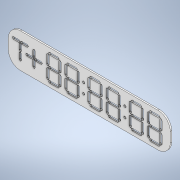
# Autodesk Inventor part: 7 Segment Clock
Saved by Autodesk Inventor 2021 (Build 250183000, 183)
## iProperties
Created: 2020-06-26
Part Number: 7 Segment Clock
Material: White
Document SubType Name: Modeling
Designer: dech3
Density: 1.188 g/cm^3
Appearance: Polycarbonate - Clear
Author: dech3
Autodesk Inventor part; units mm, degrees
(part 1 of 3)
ref_plane "YZ Plane" through (0, 0, 0) normal (1, 0, 0) x (0, 1, 0)
ref_plane "XZ Plane" through (0, 0, 0) normal (0, 1, 0) x (-1, 0, 0)
ref_plane "XY Plane" through (0, 0, 0) normal (0, 0, 1) x (1, 0, 0)
sketch "Single Segment" plane through (0, 0, 0) normal (0, 0, 1) x (1, 0, 0)
  arc A0 (128.9839, -2.0293) -> (129.691, -2.3222) centre (129.691, -1.3222) ccw
  arc A1 (129.691, 2.6778) -> (128.9839, 2.3849) centre (129.691, 1.6778) ccw
  line L0 (128.9839, -2.0293) -> (127.0768, -0.1222)
  line L1 (128.9839, 2.3849) -> (127.0768, 0.4778)
  line L2 (127.0768, 0.1778) -> (127.0768, -0.1222)
  line L3 (127.0768, 0.1778) -> (127.0768, 0.4778)
  line L4 (129.691, 2.6778) -> (146.4626, 2.6778)
  line L5 (146.4626, -2.3222) -> (129.691, -2.3222)
  arc A2 (147.1697, 2.3849) -> (146.4626, 2.6778) centre (146.4626, 1.6778) ccw
  line L6 (147.1697, 2.3849) -> (149.0768, 0.4778)
  line L7 (149.0768, 0.1778) -> (149.0768, 0.4778)
  line L8 (149.0768, 0.1778) -> (149.0768, -0.1222)
  arc A3 (146.4626, -2.3222) -> (147.1697, -2.0293) centre (146.4626, -1.3222) ccw
  line L9 (147.1697, -2.0293) -> (149.0768, -0.1222)
  point P0 (153.0768, 0)
  point P1 (129.2768, -2.3222)
  point P2 (129.2768, 2.6778)
  point P3 (146.8768, 2.6778)
  point P4 (146.8768, -2.3222)
  dimension "d105" = 2.2
  dimension "d108" = 2.2
  dimension "d111" = 2.2
  dimension "d112" = 2.2
  dimension "d113" = 2.2
  dimension "d114" = 2.2
  dimension "d115" = 2.2
  dimension "d116" = 1
  dimension "d117" = 5
  dimension "d121" = 2.2
  dimension "d122" = 2.2
  dimension "d126" = 135
  dimension "d127" = 22
  dimension "d128" = 135
  dimension "d129" = 2.5
  dimension "d348" = 5
  dimension "d349" = 22
  dimension "d350" = 2.2
  dimension "d352" = 0.3
  dimension "d353" = 0.3
  dimension "d358" = 0.3
  dimension "d359" = 0.3
  measures "d105" horizontal distance of point (129.277, -2.322) L0.end
  measures "d108" horizontal distance of L7.end point (146.877, 2.678)
  measures "d111" horizontal distance of point (129.277, 2.678) L3.end
  measures "d112" horizontal distance of L9.end point (146.877, -2.322)
  measures "d113" horizontal distance of L9.end point (146.877, -2.322)
  measures "d114" horizontal distance of point (129.277, 2.678) L3.end
  measures "d115" horizontal distance of point (129.277, -2.322) L0.end
  measures "d116" radius of A1
  measures "d117" distance of point (146.877, -2.322) point (146.877, 2.678)
  measures "d121" horizontal distance of L7.end point (146.877, 2.678)
  measures "d122" horizontal distance of point (146.877, -2.322) L8.start
  measures "d126" angle of L5 L9
  measures "d127" horizontal distance of L9.end L3.start
  measures "d128" angle of L4 L6
  measures "d129" vertical distance of L8.start point (146.877, -2.322)
  measures "d348" distance between parallel lines of L5 L4
  measures "d349" distance of L3.start L8.start
  measures "d350" horizontal distance of point (129.277, 2.678) L3.start
  measures "d352" distance of L8.start L7.end
  measures "d353" distance of L9.end L8.start
  measures "d358" distance of L3.end L3.start
  measures "d359" distance of L0.end L3.start
sketch "7 Segment Digit" plane through (0, 0, 0) normal (0, 0, 1) x (1, 0, 0)
  arc A0 (215.9071, -11.0293) -> (216.6142, -11.3222) centre (216.6142, -10.3222) ccw
  arc A1 (216.6142, -6.3222) -> (215.9071, -6.6151) centre (216.6142, -7.3222) ccw
  line L0 (215.9071, -11.0293) -> (214, -9.1222)
  line L1 (215.9071, -6.6151) -> (214, -8.5222)
  line L2 (214, -8.8222) -> (214, -9.1222)
  line L3 (214, -8.8222) -> (214, -8.5222)
  line L4 (216.6142, -6.3222) -> (233.3858, -6.3222)
  line L5 (233.3858, -11.3222) -> (216.6142, -11.3222)
  arc A2 (234.0929, -6.6151) -> (233.3858, -6.3222) centre (233.3858, -7.3222) ccw
  line L6 (234.0929, -6.6151) -> (236, -8.5222)
  line L7 (236, -8.8222) -> (236, -8.5222)
  line L8 (236, -8.8222) -> (236, -9.1222)
  arc A3 (233.3858, -11.3222) -> (234.0929, -11.0293) centre (233.3858, -10.3222) ccw
  line L9 (234.0929, -11.0293) -> (236, -9.1222)
  arc A4 (215.9071, -35.8293) -> (216.6142, -36.1222) centre (216.6142, -35.1222) ccw
  arc A5 (216.6142, -31.1222) -> (215.9071, -31.4151) centre (216.6142, -32.1222) ccw
  line L10 (215.9071, -35.8293) -> (214, -33.9222)
  line L11 (215.9071, -31.4151) -> (214, -33.3222)
  line L12 (214, -33.6222) -> (214, -33.9222)
  line L13 (214, -33.6222) -> (214, -33.3222)
  line L14 (216.6142, -31.1222) -> (233.3858, -31.1222)
  line L15 (233.3858, -36.1222) -> (216.6142, -36.1222)
  arc A6 (234.0929, -31.4151) -> (233.3858, -31.1222) centre (233.3858, -32.1222) ccw
  line L16 (234.0929, -31.4151) -> (236, -33.3222)
  line L17 (236, -33.6222) -> (236, -33.3222)
  line L18 (236, -33.6222) -> (236, -33.9222)
  arc A7 (233.3858, -36.1222) -> (234.0929, -35.8293) centre (233.3858, -35.1222) ccw
  line L19 (234.0929, -35.8293) -> (236, -33.9222)
  arc A8 (214.8071, -30.3151) -> (215.1, -29.608) centre (214.1, -29.608) ccw
  arc A9 (210.1, -29.608) -> (210.3929, -30.3151) centre (211.1, -29.608) ccw
  line L20 (214.8071, -30.3151) -> (212.9, -32.2222)
  line L21 (210.3929, -30.3151) -> (212.3, -32.2222)
  line L22 (212.6, -32.2222) -> (212.9, -32.2222)
  line L23 (212.6, -32.2222) -> (212.3, -32.2222)
  line L24 (210.1, -29.608) -> (210.1, -12.8364)
  line L25 (215.1, -12.8364) -> (215.1, -29.608)
  arc A10 (210.3929, -12.1293) -> (210.1, -12.8364) centre (211.1, -12.8364) ccw
  line L26 (210.3929, -12.1293) -> (212.3, -10.2222)
  line L27 (212.6, -10.2222) -> (212.3, -10.2222)
  line L28 (212.6, -10.2222) -> (212.9, -10.2222)
  arc A11 (215.1, -12.8364) -> (214.8071, -12.1293) centre (214.1, -12.8364) ccw
  line L29 (214.8071, -12.1293) -> (212.9, -10.2222)
  arc A12 (214.8071, -55.1151) -> (215.1, -54.408) centre (214.1, -54.408) ccw
  arc A13 (210.1, -54.408) -> (210.3929, -55.1151) centre (211.1, -54.408) ccw
  line L30 (214.8071, -55.1151) -> (212.9, -57.0222)
  line L31 (210.3929, -55.1151) -> (212.3, -57.0222)
  line L32 (212.6, -57.0222) -> (212.9, -57.0222)
  line L33 (212.6, -57.0222) -> (212.3, -57.0222)
  line L34 (210.1, -54.408) -> (210.1, -37.6364)
  line L35 (215.1, -37.6364) -> (215.1, -54.408)
  arc A14 (210.3929, -36.9293) -> (210.1, -37.6364) centre (211.1, -37.6364) ccw
  line L36 (210.3929, -36.9293) -> (212.3, -35.0222)
  line L37 (212.6, -35.0222) -> (212.3, -35.0222)
  line L38 (212.6, -35.0222) -> (212.9, -35.0222)
  arc A15 (215.1, -37.6364) -> (214.8071, -36.9293) centre (214.1, -37.6364) ccw
  line L39 (214.8071, -36.9293) -> (212.9, -35.0222)
  arc A16 (239.6071, -30.3151) -> (239.9, -29.608) centre (238.9, -29.608) ccw
  arc A17 (234.9, -29.608) -> (235.1929, -30.3151) centre (235.9, -29.608) ccw
  line L40 (239.6071, -30.3151) -> (237.7, -32.2222)
  line L41 (235.1929, -30.3151) -> (237.1, -32.2222)
  line L42 (237.4, -32.2222) -> (237.7, -32.2222)
  line L43 (237.4, -32.2222) -> (237.1, -32.2222)
  line L44 (234.9, -29.608) -> (234.9, -12.8364)
  line L45 (239.9, -12.8364) -> (239.9, -29.608)
  arc A18 (235.1929, -12.1293) -> (234.9, -12.8364) centre (235.9, -12.8364) ccw
  line L46 (235.1929, -12.1293) -> (237.1, -10.2222)
  line L47 (237.4, -10.2222) -> (237.1, -10.2222)
  line L48 (237.4, -10.2222) -> (237.7, -10.2222)
  arc A19 (239.9, -12.8364) -> (239.6071, -12.1293) centre (238.9, -12.8364) ccw
  line L49 (239.6071, -12.1293) -> (237.7, -10.2222)
  arc A20 (239.6071, -55.1151) -> (239.9, -54.408) centre (238.9, -54.408) ccw
  arc A21 (234.9, -54.408) -> (235.1929, -55.1151) centre (235.9, -54.408) ccw
  line L50 (239.6071, -55.1151) -> (237.7, -57.0222)
  line L51 (235.1929, -55.1151) -> (237.1, -57.0222)
  line L52 (237.4, -57.0222) -> (237.7, -57.0222)
  line L53 (237.4, -57.0222) -> (237.1, -57.0222)
  line L54 (234.9, -54.408) -> (234.9, -37.6364)
  line L55 (239.9, -37.6364) -> (239.9, -54.408)
  arc A22 (235.1929, -36.9293) -> (234.9, -37.6364) centre (235.9, -37.6364) ccw
  line L56 (235.1929, -36.9293) -> (237.1, -35.0222)
  line L57 (237.4, -35.0222) -> (237.1, -35.0222)
  line L58 (237.4, -35.0222) -> (237.7, -35.0222)
  arc A23 (239.9, -37.6364) -> (239.6071, -36.9293) centre (238.9, -37.6364) ccw
  line L59 (239.6071, -36.9293) -> (237.7, -35.0222)
  arc A24 (215.9071, -60.6293) -> (216.6142, -60.9222) centre (216.6142, -59.9222) ccw
  arc A25 (216.6142, -55.9222) -> (215.9071, -56.2151) centre (216.6142, -56.9222) ccw
  line L60 (215.9071, -60.6293) -> (214, -58.7222)
  line L61 (215.9071, -56.2151) -> (214, -58.1222)
  line L62 (214, -58.4222) -> (214, -58.7222)
  line L63 (214, -58.4222) -> (214, -58.1222)
  line L64 (216.6142, -55.9222) -> (233.3858, -55.9222)
  line L65 (233.3858, -60.9222) -> (216.6142, -60.9222)
  arc A26 (234.0929, -56.2151) -> (233.3858, -55.9222) centre (233.3858, -56.9222) ccw
  line L66 (234.0929, -56.2151) -> (236, -58.1222)
  line L67 (236, -58.4222) -> (236, -58.1222)
  line L68 (236, -58.4222) -> (236, -58.7222)
  arc A27 (233.3858, -60.9222) -> (234.0929, -60.6293) centre (233.3858, -59.9222) ccw
  line L69 (234.0929, -60.6293) -> (236, -58.7222)
  point P0 (239.8857, -4.9143)
  dimension "d131" = 1.1
  dimension "d132" = 1.1
  dimension "d137" = 1.1
  dimension "d138" = 1.1
  dimension "d139" = 1.1
  dimension "d140" = 1.1
  dimension "d141" = 1.1
  dimension "d142" = 1.1
  dimension "d143" = 1.1
  dimension "d144" = 1.1
  dimension "d145" = 1.1
  dimension "d146" = 1.1
  dimension "d150" = 1.1
  dimension "d151" = 1.1
  dimension "d152" = 1.1
  dimension "d153" = 1.1
sketch "Slanted Segment Large" plane through (0, 0, 0) normal (0, 0, 1) x (1, 0, 0)
  line L0 (-252.8296, -124.6537) -> (-254.4296, -124.6537)
  line L1 (-254.4296, -124.6537) -> (-257.6296, -127.8537)
  line L2 (-257.6296, -127.8537) -> (-261.6917, -184.8537)
  line L3 (-253.6917, -184.8537) -> (-249.6296, -127.8537)
  line L4 (-249.6296, -127.8537) -> (-252.8296, -124.6537)
  line L5 (-261.6917, -184.8537) -> (-258.4917, -188.0537)
  line L6 (-258.4917, -188.0537) -> (-256.8917, -188.0537)
  line L7 (-256.8917, -188.0537) -> (-253.6917, -184.8537)
  point P0 (-253.3255, -154.094)
  point P1 (-253.6296, -124.6537)
  dimension "d294" = 3.2
  dimension "d295" = 3.2
  dimension "d296" = 8
  dimension "d297" = 3.2
  dimension "d298" = 3.2
  dimension "d299" = 57
  dimension "d304" = 3.2
  dimension "d305" = 3.2
  dimension "d306" = 3.2
  dimension "d307" = 3.2
  measures "d294" horizontal distance of L0.end L1.end
  measures "d295" horizontal distance of L3.end L0.start
  measures "d296" distance of L3.end L1.end
  measures "d297" horizontal distance of L3.end L0.start
  measures "d298" horizontal distance of L0.end L1.end
  measures "d299" vertical distance of L3.end L3.start
  measures "d304" horizontal distance of L5.end L2.end
  measures "d305" horizontal distance of L3.start L6.end
  measures "d306" horizontal distance of L2.end L5.end
  measures "d307" horizontal distance of L3.start L6.end
sketch "+ sign" plane through (0, 0, 0) normal (0, 0, 1) x (1, 0, 0)
  arc A0 (1.761, -2.8041) -> (2.4681, -3.097) centre (2.4681, -2.097) ccw
  arc A1 (2.4681, 1.903) -> (1.761, 1.6102) centre (2.4681, 0.903) ccw
  line L0 (1.761, -2.8041) -> (-0.1461, -0.897)
  line L1 (-0.1461, -0.597) -> (-0.1461, -0.297)
  line L2 (-0.1461, -0.597) -> (-0.1461, -0.897)
  line L3 (1.761, 1.6102) -> (-0.1461, -0.297)
  line L4 (2.4681, 1.903) -> (13.2397, 1.903)
  line L5 (13.2397, -3.097) -> (2.4681, -3.097)
  arc A2 (13.9468, 1.6102) -> (13.2397, 1.903) centre (13.2397, 0.903) ccw
  arc A3 (13.2397, -3.097) -> (13.9468, -2.8041) centre (13.2397, -2.097) ccw
  line L6 (13.9468, -2.8041) -> (15.8539, -0.897)
  line L7 (15.8539, -0.597) -> (15.8539, -0.897)
  line L8 (15.8539, -0.597) -> (15.8539, -0.297)
  line L9 (13.9468, 1.6102) -> (15.8539, -0.297)
  arc A4 (1.061, 2.3102) -> (1.3539, 3.0173) centre (0.3539, 3.0173) ccw
  arc A5 (-3.6461, 3.0173) -> (-3.3532, 2.3102) centre (-2.6461, 3.0173) ccw
  line L10 (1.061, 2.3102) -> (-0.8461, 0.403)
  line L11 (-1.1461, 0.403) -> (-1.4461, 0.403)
  line L12 (-1.1461, 0.403) -> (-0.8461, 0.403)
  line L13 (-3.3532, 2.3102) -> (-1.4461, 0.403)
  line L14 (-3.6461, 3.0173) -> (-3.6461, 13.7888)
  line L15 (1.3539, 13.7888) -> (1.3539, 3.0173)
  arc A6 (-3.3532, 14.4959) -> (-3.6461, 13.7888) centre (-2.6461, 13.7888) ccw
  arc A7 (1.3539, 13.7888) -> (1.061, 14.4959) centre (0.3539, 13.7888) ccw
  line L16 (1.061, 14.4959) -> (-0.8461, 16.403)
  line L17 (-1.1461, 16.403) -> (-0.8461, 16.403)
  line L18 (-1.1461, 16.403) -> (-1.4461, 16.403)
  line L19 (-3.3532, 14.4959) -> (-1.4461, 16.403)
  arc A8 (-16.239, -2.8041) -> (-15.5319, -3.097) centre (-15.5319, -2.097) ccw
  arc A9 (-15.5319, 1.903) -> (-16.239, 1.6102) centre (-15.5319, 0.903) ccw
  line L20 (-16.239, -2.8041) -> (-18.1461, -0.897)
  line L21 (-18.1461, -0.597) -> (-18.1461, -0.297)
  line L22 (-18.1461, -0.597) -> (-18.1461, -0.897)
  line L23 (-16.239, 1.6102) -> (-18.1461, -0.297)
  line L24 (-15.5319, 1.903) -> (-4.7603, 1.903)
  line L25 (-4.7603, -3.097) -> (-15.5319, -3.097)
  arc A10 (-4.0532, 1.6102) -> (-4.7603, 1.903) centre (-4.7603, 0.903) ccw
  arc A11 (-4.7603, -3.097) -> (-4.0532, -2.8041) centre (-4.7603, -2.097) ccw
  line L26 (-4.0532, -2.8041) -> (-2.1461, -0.897)
  line L27 (-2.1461, -0.597) -> (-2.1461, -0.897)
  line L28 (-2.1461, -0.597) -> (-2.1461, -0.297)
  line L29 (-4.0532, 1.6102) -> (-2.1461, -0.297)
  arc A12 (1.061, -15.6898) -> (1.3539, -14.9827) centre (0.3539, -14.9827) ccw
  arc A13 (-3.6461, -14.9827) -> (-3.3532, -15.6898) centre (-2.6461, -14.9827) ccw
  line L30 (1.061, -15.6898) -> (-0.8461, -17.597)
  line L31 (-1.1461, -17.597) -> (-1.4461, -17.597)
  line L32 (-1.1461, -17.597) -> (-0.8461, -17.597)
  line L33 (-3.3532, -15.6898) -> (-1.4461, -17.597)
  line L34 (-3.6461, -14.9827) -> (-3.6461, -4.2112)
  line L35 (1.3539, -4.2112) -> (1.3539, -14.9827)
  arc A14 (-3.3532, -3.5041) -> (-3.6461, -4.2112) centre (-2.6461, -4.2112) ccw
  arc A15 (1.3539, -4.2112) -> (1.061, -3.5041) centre (0.3539, -4.2112) ccw
  line L36 (1.061, -3.5041) -> (-0.8461, -1.597)
  line L37 (-1.1461, -1.597) -> (-0.8461, -1.597)
  line L38 (-1.1461, -1.597) -> (-1.4461, -1.597)
  line L39 (-3.3532, -3.5041) -> (-1.4461, -1.597)
  point P0 (-225.4266, -6.7349)
  dimension "d496" = 2
  dimension "d497" = 2
  dimension "d501" = 1
  dimension "d502" = 1
  dimension "d503" = 0
  dimension "d504" = 0
  dimension "d505" = 0.99
  dimension "d506" = 0.99
  dimension "d507" = 0.99
  dimension "d508" = 0.99
sketch "Dot" plane through (0, 0, 0) normal (0, 0, 1) x (1, 0, 0)
  line L0 (-36.1663, 28.3091) -> (-35.1663, 28.3091)
  line L1 (-35.1663, 28.3091) -> (-33.1663, 26.3091)
  line L2 (-33.1663, 26.3091) -> (-33.1663, 25.3091)
  line L3 (-33.1663, 25.3091) -> (-35.1663, 23.3091)
  line L4 (-35.1663, 23.3091) -> (-36.1663, 23.3091)
  line L5 (-36.1663, 23.3091) -> (-38.1663, 25.3091)
  line L6 (-38.1663, 25.3091) -> (-38.1663, 26.3091)
  line L7 (-38.1663, 26.3091) -> (-36.1663, 28.3091)
  point P0 (-33.9663, 25.3091)
  dimension "d311" = 2
  dimension "d312" = 2
  dimension "d314" = 2
  dimension "d315" = 2
  dimension "d316" = 2
  dimension "d317" = 2
  dimension "d318" = 2
  dimension "d319" = 2
  dimension "d320" = 1
  dimension "d321" = 1
  dimension "d322" = 1
  dimension "d323" = 1
  dimension "d360" = 5
  dimension "d361" = 5
  measures "d311" horizontal distance of L1.end L0.end
  measures "d312" horizontal distance of L0.start L6.end
  measures "d314" horizontal distance of L0.start L6.end
  measures "d315" horizontal distance of L1.end L0.end
  measures "d316" horizontal distance of L4.end L5.end
  measures "d317" horizontal distance of L2.end L3.end
  measures "d318" horizontal distance of L2.end L3.end
  measures "d319" horizontal distance of L5.end L4.end
  measures "d320" distance of L1.end L2.end
  measures "d321" distance of L0.end L0.start
  measures "d322" distance of L3.end L4.end
  measures "d323" distance of L6.end L5.end
  measures "d360" distance between parallel lines of L4 L0
  measures "d361" distance between parallel lines of L2 L6
sketch "Clock Face with T +-" plane through (0, 0, 0) normal (0, 0, 1) x (1, 0, 0)
  arc A0 (55.0672, 19.3353) -> (55.7743, 19.0424) centre (55.7743, 20.0424) ccw
  arc A1 (55.7743, 24.0424) -> (55.0672, 23.7495) centre (55.7743, 23.0424) ccw
  line L0 (55.0672, 19.3353) -> (53.1601, 21.2424)
  line L1 (55.0672, 23.7495) -> (53.1601, 21.8424)
  line L2 (53.1601, 21.5424) -> (53.1601, 21.2424)
  line L3 (53.1601, 21.5424) -> (53.1601, 21.8424)
  line L4 (55.7743, 24.0424) -> (72.5459, 24.0424)
  line L5 (72.5459, 19.0424) -> (55.7743, 19.0424)
  arc A2 (73.253, 23.7495) -> (72.5459, 24.0424) centre (72.5459, 23.0424) ccw
  line L6 (73.253, 23.7495) -> (75.1601, 21.8424)
  line L7 (75.1601, 21.5424) -> (75.1601, 21.8424)
  line L8 (75.1601, 21.5424) -> (75.1601, 21.2424)
  arc A3 (72.5459, 19.0424) -> (73.253, 19.3353) centre (72.5459, 20.0424) ccw
  line L9 (73.253, 19.3353) -> (75.1601, 21.2424)
  arc A4 (55.0672, -5.4647) -> (55.7743, -5.7576) centre (55.7743, -4.7576) ccw
  arc A5 (55.7743, -0.7576) -> (55.0672, -1.0505) centre (55.7743, -1.7576) ccw
  line L10 (55.0672, -5.4647) -> (53.1601, -3.5576)
  line L11 (55.0672, -1.0505) -> (53.1601, -2.9576)
  line L12 (53.1601, -3.2576) -> (53.1601, -3.5576)
  line L13 (53.1601, -3.2576) -> (53.1601, -2.9576)
  line L14 (55.7743, -0.7576) -> (72.5459, -0.7576)
  line L15 (72.5459, -5.7576) -> (55.7743, -5.7576)
  arc A6 (73.253, -1.0505) -> (72.5459, -0.7576) centre (72.5459, -1.7576) ccw
  line L16 (73.253, -1.0505) -> (75.1601, -2.9576)
  line L17 (75.1601, -3.2576) -> (75.1601, -2.9576)
  line L18 (75.1601, -3.2576) -> (75.1601, -3.5576)
  arc A7 (72.5459, -5.7576) -> (73.253, -5.4647) centre (72.5459, -4.7576) ccw
  line L19 (73.253, -5.4647) -> (75.1601, -3.5576)
  arc A8 (53.9672, 0.0495) -> (54.2601, 0.7566) centre (53.2601, 0.7566) ccw
  arc A9 (49.2601, 0.7566) -> (49.553, 0.0495) centre (50.2601, 0.7566) ccw
  line L20 (53.9672, 0.0495) -> (52.0601, -1.8576)
  line L21 (49.553, 0.0495) -> (51.4601, -1.8576)
  line L22 (51.7601, -1.8576) -> (52.0601, -1.8576)
  line L23 (51.7601, -1.8576) -> (51.4601, -1.8576)
  line L24 (49.2601, 0.7566) -> (49.2601, 17.5282)
  line L25 (54.2601, 17.5282) -> (54.2601, 0.7566)
  arc A10 (49.553, 18.2353) -> (49.2601, 17.5282) centre (50.2601, 17.5282) ccw
  line L26 (49.553, 18.2353) -> (51.4601, 20.1424)
  line L27 (51.7601, 20.1424) -> (51.4601, 20.1424)
  line L28 (51.7601, 20.1424) -> (52.0601, 20.1424)
  arc A11 (54.2601, 17.5282) -> (53.9672, 18.2353) centre (53.2601, 17.5282) ccw
  line L29 (53.9672, 18.2353) -> (52.0601, 20.1424)
  arc A12 (53.9672, -24.7505) -> (54.2601, -24.0434) centre (53.2601, -24.0434) ccw
  arc A13 (49.2601, -24.0434) -> (49.553, -24.7505) centre (50.2601, -24.0434) ccw
  line L30 (53.9672, -24.7505) -> (52.0601, -26.6576)
  line L31 (49.553, -24.7505) -> (51.4601, -26.6576)
  line L32 (51.7601, -26.6576) -> (52.0601, -26.6576)
  line L33 (51.7601, -26.6576) -> (51.4601, -26.6576)
  line L34 (49.2601, -24.0434) -> (49.2601, -7.2718)
  line L35 (54.2601, -7.2718) -> (54.2601, -24.0434)
  arc A14 (49.553, -6.5647) -> (49.2601, -7.2718) centre (50.2601, -7.2718) ccw
  line L36 (49.553, -6.5647) -> (51.4601, -4.6576)
  line L37 (51.7601, -4.6576) -> (51.4601, -4.6576)
  line L38 (51.7601, -4.6576) -> (52.0601, -4.6576)
  arc A15 (54.2601, -7.2718) -> (53.9672, -6.5647) centre (53.2601, -7.2718) ccw
  line L39 (53.9672, -6.5647) -> (52.0601, -4.6576)
  arc A16 (78.7672, 0.0495) -> (79.0601, 0.7566) centre (78.0601, 0.7566) ccw
  arc A17 (74.0601, 0.7566) -> (74.353, 0.0495) centre (75.0601, 0.7566) ccw
  line L40 (78.7672, 0.0495) -> (76.8601, -1.8576)
  line L41 (74.353, 0.0495) -> (76.2601, -1.8576)
  line L42 (76.5601, -1.8576) -> (76.8601, -1.8576)
  line L43 (76.5601, -1.8576) -> (76.2601, -1.8576)
  line L44 (74.0601, 0.7566) -> (74.0601, 17.5282)
  line L45 (79.0601, 17.5282) -> (79.0601, 0.7566)
  arc A18 (74.353, 18.2353) -> (74.0601, 17.5282) centre (75.0601, 17.5282) ccw
  line L46 (74.353, 18.2353) -> (76.2601, 20.1424)
  line L47 (76.5601, 20.1424) -> (76.2601, 20.1424)
  line L48 (76.5601, 20.1424) -> (76.8601, 20.1424)
  arc A19 (79.0601, 17.5282) -> (78.7672, 18.2353) centre (78.0601, 17.5282) ccw
  line L49 (78.7672, 18.2353) -> (76.8601, 20.1424)
  arc A20 (78.7672, -24.7505) -> (79.0601, -24.0434) centre (78.0601, -24.0434) ccw
  arc A21 (74.0601, -24.0434) -> (74.353, -24.7505) centre (75.0601, -24.0434) ccw
  line L50 (78.7672, -24.7505) -> (76.8601, -26.6576)
  line L51 (74.353, -24.7505) -> (76.2601, -26.6576)
  line L52 (76.5601, -26.6576) -> (76.8601, -26.6576)
  line L53 (76.5601, -26.6576) -> (76.2601, -26.6576)
  line L54 (74.0601, -24.0434) -> (74.0601, -7.2718)
  line L55 (79.0601, -7.2718) -> (79.0601, -24.0434)
  arc A22 (74.353, -6.5647) -> (74.0601, -7.2718) centre (75.0601, -7.2718) ccw
  line L56 (74.353, -6.5647) -> (76.2601, -4.6576)
  line L57 (76.5601, -4.6576) -> (76.2601, -4.6576)
  line L58 (76.5601, -4.6576) -> (76.8601, -4.6576)
  arc A23 (79.0601, -7.2718) -> (78.7672, -6.5647) centre (78.0601, -7.2718) ccw
  line L59 (78.7672, -6.5647) -> (76.8601, -4.6576)
  arc A24 (55.0672, -30.2647) -> (55.7743, -30.5576) centre (55.7743, -29.5576) ccw
  arc A25 (55.7743, -25.5576) -> (55.0672, -25.8505) centre (55.7743, -26.5576) ccw
  line L60 (55.0672, -30.2647) -> (53.1601, -28.3576)
  line L61 (55.0672, -25.8505) -> (53.1601, -27.7576)
  line L62 (53.1601, -28.0576) -> (53.1601, -28.3576)
  line L63 (53.1601, -28.0576) -> (53.1601, -27.7576)
  line L64 (55.7743, -25.5576) -> (72.5459, -25.5576)
  line L65 (72.5459, -30.5576) -> (55.7743, -30.5576)
  arc A26 (73.253, -25.8505) -> (72.5459, -25.5576) centre (72.5459, -26.5576) ccw
  line L66 (73.253, -25.8505) -> (75.1601, -27.7576)
  line L67 (75.1601, -28.0576) -> (75.1601, -27.7576)
  line L68 (75.1601, -28.0576) -> (75.1601, -28.3576)
  arc A27 (72.5459, -30.5576) -> (73.253, -30.2647) centre (72.5459, -29.5576) ccw
  line L69 (73.253, -30.2647) -> (75.1601, -28.3576)
  arc A28 (8.2672, 19.3353) -> (8.9743, 19.0424) centre (8.9743, 20.0424) ccw
  arc A29 (8.9743, 24.0424) -> (8.2672, 23.7495) centre (8.9743, 23.0424) ccw
  line L70 (8.2672, 19.3353) -> (6.3601, 21.2424)
  line L71 (8.2672, 23.7495) -> (6.3601, 21.8424)
  line L72 (6.3601, 21.5424) -> (6.3601, 21.2424)
  line L73 (6.3601, 21.5424) -> (6.3601, 21.8424)
  line L74 (8.9743, 24.0424) -> (25.7459, 24.0424)
  line L75 (25.7459, 19.0424) -> (8.9743, 19.0424)
  arc A30 (26.453, 23.7495) -> (25.7459, 24.0424) centre (25.7459, 23.0424) ccw
  line L76 (26.453, 23.7495) -> (28.3601, 21.8424)
  line L77 (28.3601, 21.5424) -> (28.3601, 21.8424)
  line L78 (28.3601, 21.5424) -> (28.3601, 21.2424)
  arc A31 (25.7459, 19.0424) -> (26.453, 19.3353) centre (25.7459, 20.0424) ccw
  line L79 (26.453, 19.3353) -> (28.3601, 21.2424)
  arc A32 (8.2672, -5.4647) -> (8.9743, -5.7576) centre (8.9743, -4.7576) ccw
  arc A33 (8.9743, -0.7576) -> (8.2672, -1.0505) centre (8.9743, -1.7576) ccw
  line L80 (8.2672, -5.4647) -> (6.3601, -3.5576)
  line L81 (8.2672, -1.0505) -> (6.3601, -2.9576)
  line L82 (6.3601, -3.2576) -> (6.3601, -3.5576)
  line L83 (6.3601, -3.2576) -> (6.3601, -2.9576)
  line L84 (8.9743, -0.7576) -> (25.7459, -0.7576)
  line L85 (25.7459, -5.7576) -> (8.9743, -5.7576)
  arc A34 (26.453, -1.0505) -> (25.7459, -0.7576) centre (25.7459, -1.7576) ccw
  line L86 (26.453, -1.0505) -> (28.3601, -2.9576)
  line L87 (28.3601, -3.2576) -> (28.3601, -2.9576)
  line L88 (28.3601, -3.2576) -> (28.3601, -3.5576)
  arc A35 (25.7459, -5.7576) -> (26.453, -5.4647) centre (25.7459, -4.7576) ccw
  line L89 (26.453, -5.4647) -> (28.3601, -3.5576)
  arc A36 (7.1672, 0.0495) -> (7.4601, 0.7566) centre (6.4601, 0.7566) ccw
  arc A37 (2.4601, 0.7566) -> (2.753, 0.0495) centre (3.4601, 0.7566) ccw
  line L90 (7.1672, 0.0495) -> (5.2601, -1.8576)
  line L91 (2.753, 0.0495) -> (4.6601, -1.8576)
  line L92 (4.9601, -1.8576) -> (5.2601, -1.8576)
  line L93 (4.9601, -1.8576) -> (4.6601, -1.8576)
  line L94 (2.4601, 0.7566) -> (2.4601, 17.5282)
  line L95 (7.4601, 17.5282) -> (7.4601, 0.7566)
  arc A38 (2.753, 18.2353) -> (2.4601, 17.5282) centre (3.4601, 17.5282) ccw
  line L96 (2.753, 18.2353) -> (4.6601, 20.1424)
  line L97 (4.9601, 20.1424) -> (4.6601, 20.1424)
  line L98 (4.9601, 20.1424) -> (5.2601, 20.1424)
  arc A39 (7.4601, 17.5282) -> (7.1672, 18.2353) centre (6.4601, 17.5282) ccw
  line L99 (7.1672, 18.2353) -> (5.2601, 20.1424)
  arc A40 (7.1672, -24.7505) -> (7.4601, -24.0434) centre (6.4601, -24.0434) ccw
  arc A41 (2.4601, -24.0434) -> (2.753, -24.7505) centre (3.4601, -24.0434) ccw
  line L100 (7.1672, -24.7505) -> (5.2601, -26.6576)
  line L101 (2.753, -24.7505) -> (4.6601, -26.6576)
  line L102 (4.9601, -26.6576) -> (5.2601, -26.6576)
  line L103 (4.9601, -26.6576) -> (4.6601, -26.6576)
  line L104 (2.4601, -24.0434) -> (2.4601, -7.2718)
  line L105 (7.4601, -7.2718) -> (7.4601, -24.0434)
  arc A42 (2.753, -6.5647) -> (2.4601, -7.2718) centre (3.4601, -7.2718) ccw
  line L106 (2.753, -6.5647) -> (4.6601, -4.6576)
  line L107 (4.9601, -4.6576) -> (4.6601, -4.6576)
  line L108 (4.9601, -4.6576) -> (5.2601, -4.6576)
  arc A43 (7.4601, -7.2718) -> (7.1672, -6.5647) centre (6.4601, -7.2718) ccw
  line L109 (7.1672, -6.5647) -> (5.2601, -4.6576)
  arc A44 (31.9672, 0.0495) -> (32.2601, 0.7566) centre (31.2601, 0.7566) ccw
  arc A45 (27.2601, 0.7566) -> (27.553, 0.0495) centre (28.2601, 0.7566) ccw
  line L110 (31.9672, 0.0495) -> (30.0601, -1.8576)
  line L111 (27.553, 0.0495) -> (29.4601, -1.8576)
  line L112 (29.7601, -1.8576) -> (30.0601, -1.8576)
  line L113 (29.7601, -1.8576) -> (29.4601, -1.8576)
  line L114 (27.2601, 0.7566) -> (27.2601, 17.5282)
  line L115 (32.2601, 17.5282) -> (32.2601, 0.7566)
  arc A46 (27.553, 18.2353) -> (27.2601, 17.5282) centre (28.2601, 17.5282) ccw
  line L116 (27.553, 18.2353) -> (29.4601, 20.1424)
  line L117 (29.7601, 20.1424) -> (29.4601, 20.1424)
  line L118 (29.7601, 20.1424) -> (30.0601, 20.1424)
  arc A47 (32.2601, 17.5282) -> (31.9672, 18.2353) centre (31.2601, 17.5282) ccw
  line L119 (31.9672, 18.2353) -> (30.0601, 20.1424)
  arc A48 (31.9672, -24.7505) -> (32.2601, -24.0434) centre (31.2601, -24.0434) ccw
  arc A49 (27.2601, -24.0434) -> (27.553, -24.7505) centre (28.2601, -24.0434) ccw
  line L120 (31.9672, -24.7505) -> (30.0601, -26.6576)
  line L121 (27.553, -24.7505) -> (29.4601, -26.6576)
  line L122 (29.7601, -26.6576) -> (30.0601, -26.6576)
  line L123 (29.7601, -26.6576) -> (29.4601, -26.6576)
  line L124 (27.2601, -24.0434) -> (27.2601, -7.2718)
  line L125 (32.2601, -7.2718) -> (32.2601, -24.0434)
  arc A50 (27.553, -6.5647) -> (27.2601, -7.2718) centre (28.2601, -7.2718) ccw
  line L126 (27.553, -6.5647) -> (29.4601, -4.6576)
  line L127 (29.7601, -4.6576) -> (29.4601, -4.6576)
  line L128 (29.7601, -4.6576) -> (30.0601, -4.6576)
  arc A51 (32.2601, -7.2718) -> (31.9672, -6.5647) centre (31.2601, -7.2718) ccw
  line L129 (31.9672, -6.5647) -> (30.0601, -4.6576)
  arc A52 (8.2672, -30.2647) -> (8.9743, -30.5576) centre (8.9743, -29.5576) ccw
  arc A53 (8.9743, -25.5576) -> (8.2672, -25.8505) centre (8.9743, -26.5576) ccw
  line L130 (8.2672, -30.2647) -> (6.3601, -28.3576)
  line L131 (8.2672, -25.8505) -> (6.3601, -27.7576)
  line L132 (6.3601, -28.0576) -> (6.3601, -28.3576)
  line L133 (6.3601, -28.0576) -> (6.3601, -27.7576)
  line L134 (8.9743, -25.5576) -> (25.7459, -25.5576)
  line L135 (25.7459, -30.5576) -> (8.9743, -30.5576)
  arc A54 (26.453, -25.8505) -> (25.7459, -25.5576) centre (25.7459, -26.5576) ccw
  line L136 (26.453, -25.8505) -> (28.3601, -27.7576)
  line L137 (28.3601, -28.0576) -> (28.3601, -27.7576)
  line L138 (28.3601, -28.0576) -> (28.3601, -28.3576)
  arc A55 (25.7459, -30.5576) -> (26.453, -30.2647) centre (25.7459, -29.5576) ccw
  line L139 (26.453, -30.2647) -> (28.3601, -28.3576)
  arc A56 (-29.0328, 19.3353) -> (-28.3257, 19.0424) centre (-28.3257, 20.0424) ccw
  arc A57 (-28.3257, 24.0424) -> (-29.0328, 23.7495) centre (-28.3257, 23.0424) ccw
  line L140 (-29.0328, 19.3353) -> (-30.9399, 21.2424)
  line L141 (-29.0328, 23.7495) -> (-30.9399, 21.8424)
  line L142 (-30.9399, 21.5424) -> (-30.9399, 21.2424)
  line L143 (-30.9399, 21.5424) -> (-30.9399, 21.8424)
  line L144 (-28.3257, 24.0424) -> (-11.5541, 24.0424)
  line L145 (-11.5541, 19.0424) -> (-28.3257, 19.0424)
  arc A58 (-10.847, 23.7495) -> (-11.5541, 24.0424) centre (-11.5541, 23.0424) ccw
  line L146 (-10.847, 23.7495) -> (-8.9399, 21.8424)
  line L147 (-8.9399, 21.5424) -> (-8.9399, 21.8424)
  line L148 (-8.9399, 21.5424) -> (-8.9399, 21.2424)
  arc A59 (-11.5541, 19.0424) -> (-10.847, 19.3353) centre (-11.5541, 20.0424) ccw
  line L149 (-10.847, 19.3353) -> (-8.9399, 21.2424)
  arc A60 (-29.0328, -5.4647) -> (-28.3257, -5.7576) centre (-28.3257, -4.7576) ccw
  arc A61 (-28.3257, -0.7576) -> (-29.0328, -1.0505) centre (-28.3257, -1.7576) ccw
  line L150 (-29.0328, -5.4647) -> (-30.9399, -3.5576)
  line L151 (-29.0328, -1.0505) -> (-30.9399, -2.9576)
  line L152 (-30.9399, -3.2576) -> (-30.9399, -3.5576)
  line L153 (-30.9399, -3.2576) -> (-30.9399, -2.9576)
  line L154 (-28.3257, -0.7576) -> (-11.5541, -0.7576)
  line L155 (-11.5541, -5.7576) -> (-28.3257, -5.7576)
  arc A62 (-10.847, -1.0505) -> (-11.5541, -0.7576) centre (-11.5541, -1.7576) ccw
  line L156 (-10.847, -1.0505) -> (-8.9399, -2.9576)
  line L157 (-8.9399, -3.2576) -> (-8.9399, -2.9576)
  line L158 (-8.9399, -3.2576) -> (-8.9399, -3.5576)
  arc A63 (-11.5541, -5.7576) -> (-10.847, -5.4647) centre (-11.5541, -4.7576) ccw
  line L159 (-10.847, -5.4647) -> (-8.9399, -3.5576)
  arc A64 (-30.1328, 0.0495) -> (-29.8399, 0.7566) centre (-30.8399, 0.7566) ccw
  arc A65 (-34.8399, 0.7566) -> (-34.547, 0.0495) centre (-33.8399, 0.7566) ccw
  line L160 (-30.1328, 0.0495) -> (-32.0399, -1.8576)
  line L161 (-34.547, 0.0495) -> (-32.6399, -1.8576)
  line L162 (-32.3399, -1.8576) -> (-32.0399, -1.8576)
  line L163 (-32.3399, -1.8576) -> (-32.6399, -1.8576)
  line L164 (-34.8399, 0.7566) -> (-34.8399, 17.5282)
  line L165 (-29.8399, 17.5282) -> (-29.8399, 0.7566)
  arc A66 (-34.547, 18.2353) -> (-34.8399, 17.5282) centre (-33.8399, 17.5282) ccw
  line L166 (-34.547, 18.2353) -> (-32.6399, 20.1424)
  line L167 (-32.3399, 20.1424) -> (-32.6399, 20.1424)
  line L168 (-32.3399, 20.1424) -> (-32.0399, 20.1424)
  arc A67 (-29.8399, 17.5282) -> (-30.1328, 18.2353) centre (-30.8399, 17.5282) ccw
  line L169 (-30.1328, 18.2353) -> (-32.0399, 20.1424)
  arc A68 (-30.1328, -24.7505) -> (-29.8399, -24.0434) centre (-30.8399, -24.0434) ccw
  arc A69 (-34.8399, -24.0434) -> (-34.547, -24.7505) centre (-33.8399, -24.0434) ccw
  line L170 (-30.1328, -24.7505) -> (-32.0399, -26.6576)
  line L171 (-34.547, -24.7505) -> (-32.6399, -26.6576)
  line L172 (-32.3399, -26.6576) -> (-32.0399, -26.6576)
  line L173 (-32.3399, -26.6576) -> (-32.6399, -26.6576)
  line L174 (-34.8399, -24.0434) -> (-34.8399, -7.2718)
  line L175 (-29.8399, -7.2718) -> (-29.8399, -24.0434)
  arc A70 (-34.547, -6.5647) -> (-34.8399, -7.2718) centre (-33.8399, -7.2718) ccw
  line L176 (-34.547, -6.5647) -> (-32.6399, -4.6576)
  line L177 (-32.3399, -4.6576) -> (-32.6399, -4.6576)
  line L178 (-32.3399, -4.6576) -> (-32.0399, -4.6576)
  arc A71 (-29.8399, -7.2718) -> (-30.1328, -6.5647) centre (-30.8399, -7.2718) ccw
  line L179 (-30.1328, -6.5647) -> (-32.0399, -4.6576)
  arc A72 (-5.3328, 0.0495) -> (-5.0399, 0.7566) centre (-6.0399, 0.7566) ccw
  arc A73 (-10.0399, 0.7566) -> (-9.747, 0.0495) centre (-9.0399, 0.7566) ccw
  line L180 (-5.3328, 0.0495) -> (-7.2399, -1.8576)
  line L181 (-9.747, 0.0495) -> (-7.8399, -1.8576)
  line L182 (-7.5399, -1.8576) -> (-7.2399, -1.8576)
  line L183 (-7.5399, -1.8576) -> (-7.8399, -1.8576)
  line L184 (-10.0399, 0.7566) -> (-10.0399, 17.5282)
  line L185 (-5.0399, 17.5282) -> (-5.0399, 0.7566)
  arc A74 (-9.747, 18.2353) -> (-10.0399, 17.5282) centre (-9.0399, 17.5282) ccw
  line L186 (-9.747, 18.2353) -> (-7.8399, 20.1424)
  line L187 (-7.5399, 20.1424) -> (-7.8399, 20.1424)
  line L188 (-7.5399, 20.1424) -> (-7.2399, 20.1424)
  arc A75 (-5.0399, 17.5282) -> (-5.3328, 18.2353) centre (-6.0399, 17.5282) ccw
  line L189 (-5.3328, 18.2353) -> (-7.2399, 20.1424)
  arc A76 (-5.3328, -24.7505) -> (-5.0399, -24.0434) centre (-6.0399, -24.0434) ccw
  arc A77 (-10.0399, -24.0434) -> (-9.747, -24.7505) centre (-9.0399, -24.0434) ccw
  line L190 (-5.3328, -24.7505) -> (-7.2399, -26.6576)
  line L191 (-9.747, -24.7505) -> (-7.8399, -26.6576)
  line L192 (-7.5399, -26.6576) -> (-7.2399, -26.6576)
  line L193 (-7.5399, -26.6576) -> (-7.8399, -26.6576)
  line L194 (-10.0399, -24.0434) -> (-10.0399, -7.2718)
  line L195 (-5.0399, -7.2718) -> (-5.0399, -24.0434)
  arc A78 (-9.747, -6.5647) -> (-10.0399, -7.2718) centre (-9.0399, -7.2718) ccw
  line L196 (-9.747, -6.5647) -> (-7.8399, -4.6576)
  line L197 (-7.5399, -4.6576) -> (-7.8399, -4.6576)
  line L198 (-7.5399, -4.6576) -> (-7.2399, -4.6576)
  arc A79 (-5.0399, -7.2718) -> (-5.3328, -6.5647) centre (-6.0399, -7.2718) ccw
  line L199 (-5.3328, -6.5647) -> (-7.2399, -4.6576)
  arc A80 (-29.0328, -30.2647) -> (-28.3257, -30.5576) centre (-28.3257, -29.5576) ccw
  arc A81 (-28.3257, -25.5576) -> (-29.0328, -25.8505) centre (-28.3257, -26.5576) ccw
  line L200 (-29.0328, -30.2647) -> (-30.9399, -28.3576)
  line L201 (-29.0328, -25.8505) -> (-30.9399, -27.7576)
  line L202 (-30.9399, -28.0576) -> (-30.9399, -28.3576)
  line L203 (-30.9399, -28.0576) -> (-30.9399, -27.7576)
  line L204 (-28.3257, -25.5576) -> (-11.5541, -25.5576)
  line L205 (-11.5541, -30.5576) -> (-28.3257, -30.5576)
  arc A82 (-10.847, -25.8505) -> (-11.5541, -25.5576) centre (-11.5541, -26.5576) ccw
  line L206 (-10.847, -25.8505) -> (-8.9399, -27.7576)
  line L207 (-8.9399, -28.0576) -> (-8.9399, -27.7576)
  line L208 (-8.9399, -28.0576) -> (-8.9399, -28.3576)
  arc A83 (-11.5541, -30.5576) -> (-10.847, -30.2647) centre (-11.5541, -29.5576) ccw
  line L209 (-10.847, -30.2647) -> (-8.9399, -28.3576)
  arc A84 (-75.8328, 19.3353) -> (-75.1257, 19.0424) centre (-75.1257, 20.0424) ccw
  arc A85 (-75.1257, 24.0424) -> (-75.8328, 23.7495) centre (-75.1257, 23.0424) ccw
  line L210 (-75.8328, 19.3353) -> (-77.7399, 21.2424)
  line L211 (-75.8328, 23.7495) -> (-77.7399, 21.8424)
  line L212 (-77.7399, 21.5424) -> (-77.7399, 21.2424)
  line L213 (-77.7399, 21.5424) -> (-77.7399, 21.8424)
  line L214 (-75.1257, 24.0424) -> (-58.3541, 24.0424)
  line L215 (-58.3541, 19.0424) -> (-75.1257, 19.0424)
  arc A86 (-57.647, 23.7495) -> (-58.3541, 24.0424) centre (-58.3541, 23.0424) ccw
  line L216 (-57.647, 23.7495) -> (-55.7399, 21.8424)
  line L217 (-55.7399, 21.5424) -> (-55.7399, 21.8424)
  line L218 (-55.7399, 21.5424) -> (-55.7399, 21.2424)
  arc A87 (-58.3541, 19.0424) -> (-57.647, 19.3353) centre (-58.3541, 20.0424) ccw
  line L219 (-57.647, 19.3353) -> (-55.7399, 21.2424)
  arc A88 (-75.8328, -5.4647) -> (-75.1257, -5.7576) centre (-75.1257, -4.7576) ccw
  arc A89 (-75.1257, -0.7576) -> (-75.8328, -1.0505) centre (-75.1257, -1.7576) ccw
  line L220 (-75.8328, -5.4647) -> (-77.7399, -3.5576)
  line L221 (-75.8328, -1.0505) -> (-77.7399, -2.9576)
  line L222 (-77.7399, -3.2576) -> (-77.7399, -3.5576)
  line L223 (-77.7399, -3.2576) -> (-77.7399, -2.9576)
  line L224 (-75.1257, -0.7576) -> (-58.3541, -0.7576)
  line L225 (-58.3541, -5.7576) -> (-75.1257, -5.7576)
  arc A90 (-57.647, -1.0505) -> (-58.3541, -0.7576) centre (-58.3541, -1.7576) ccw
  line L226 (-57.647, -1.0505) -> (-55.7399, -2.9576)
  line L227 (-55.7399, -3.2576) -> (-55.7399, -2.9576)
  line L228 (-55.7399, -3.2576) -> (-55.7399, -3.5576)
  arc A91 (-58.3541, -5.7576) -> (-57.647, -5.4647) centre (-58.3541, -4.7576) ccw
  line L229 (-57.647, -5.4647) -> (-55.7399, -3.5576)
  arc A92 (-76.9328, 0.0495) -> (-76.6399, 0.7566) centre (-77.6399, 0.7566) ccw
  arc A93 (-81.6399, 0.7566) -> (-81.347, 0.0495) centre (-80.6399, 0.7566) ccw
  line L230 (-76.9328, 0.0495) -> (-78.8399, -1.8576)
  line L231 (-81.347, 0.0495) -> (-79.4399, -1.8576)
  line L232 (-79.1399, -1.8576) -> (-78.8399, -1.8576)
  line L233 (-79.1399, -1.8576) -> (-79.4399, -1.8576)
  line L234 (-81.6399, 0.7566) -> (-81.6399, 17.5282)
  line L235 (-76.6399, 17.5282) -> (-76.6399, 0.7566)
  arc A94 (-81.347, 18.2353) -> (-81.6399, 17.5282) centre (-80.6399, 17.5282) ccw
  line L236 (-81.347, 18.2353) -> (-79.4399, 20.1424)
  line L237 (-79.1399, 20.1424) -> (-79.4399, 20.1424)
  line L238 (-79.1399, 20.1424) -> (-78.8399, 20.1424)
  arc A95 (-76.6399, 17.5282) -> (-76.9328, 18.2353) centre (-77.6399, 17.5282) ccw
  line L239 (-76.9328, 18.2353) -> (-78.8399, 20.1424)
  arc A96 (-76.9328, -24.7505) -> (-76.6399, -24.0434) centre (-77.6399, -24.0434) ccw
  arc A97 (-81.6399, -24.0434) -> (-81.347, -24.7505) centre (-80.6399, -24.0434) ccw
  line L240 (-76.9328, -24.7505) -> (-78.8399, -26.6576)
  line L241 (-81.347, -24.7505) -> (-79.4399, -26.6576)
  line L242 (-79.1399, -26.6576) -> (-78.8399, -26.6576)
  line L243 (-79.1399, -26.6576) -> (-79.4399, -26.6576)
  line L244 (-81.6399, -24.0434) -> (-81.6399, -7.2718)
  line L245 (-76.6399, -7.2718) -> (-76.6399, -24.0434)
  arc A98 (-81.347, -6.5647) -> (-81.6399, -7.2718) centre (-80.6399, -7.2718) ccw
  line L246 (-81.347, -6.5647) -> (-79.4399, -4.6576)
  line L247 (-79.1399, -4.6576) -> (-79.4399, -4.6576)
  line L248 (-79.1399, -4.6576) -> (-78.8399, -4.6576)
  arc A99 (-76.6399, -7.2718) -> (-76.9328, -6.5647) centre (-77.6399, -7.2718) ccw
  line L249 (-76.9328, -6.5647) -> (-78.8399, -4.6576)
  arc A100 (-52.1328, 0.0495) -> (-51.8399, 0.7566) centre (-52.8399, 0.7566) ccw
  arc A101 (-56.8399, 0.7566) -> (-56.547, 0.0495) centre (-55.8399, 0.7566) ccw
  line L250 (-52.1328, 0.0495) -> (-54.0399, -1.8576)
  line L251 (-56.547, 0.0495) -> (-54.6399, -1.8576)
  line L252 (-54.3399, -1.8576) -> (-54.0399, -1.8576)
  line L253 (-54.3399, -1.8576) -> (-54.6399, -1.8576)
  line L254 (-56.8399, 0.7566) -> (-56.8399, 17.5282)
  line L255 (-51.8399, 17.5282) -> (-51.8399, 0.7566)
  arc A102 (-56.547, 18.2353) -> (-56.8399, 17.5282) centre (-55.8399, 17.5282) ccw
  line L256 (-56.547, 18.2353) -> (-54.6399, 20.1424)
  line L257 (-54.3399, 20.1424) -> (-54.6399, 20.1424)
  line L258 (-54.3399, 20.1424) -> (-54.0399, 20.1424)
  arc A103 (-51.8399, 17.5282) -> (-52.1328, 18.2353) centre (-52.8399, 17.5282) ccw
  line L259 (-52.1328, 18.2353) -> (-54.0399, 20.1424)
  arc A104 (-52.1328, -24.7505) -> (-51.8399, -24.0434) centre (-52.8399, -24.0434) ccw
  arc A105 (-56.8399, -24.0434) -> (-56.547, -24.7505) centre (-55.8399, -24.0434) ccw
  line L260 (-52.1328, -24.7505) -> (-54.0399, -26.6576)
  line L261 (-56.547, -24.7505) -> (-54.6399, -26.6576)
  line L262 (-54.3399, -26.6576) -> (-54.0399, -26.6576)
  line L263 (-54.3399, -26.6576) -> (-54.6399, -26.6576)
  line L264 (-56.8399, -24.0434) -> (-56.8399, -7.2718)
  line L265 (-51.8399, -7.2718) -> (-51.8399, -24.0434)
  arc A106 (-56.547, -6.5647) -> (-56.8399, -7.2718) centre (-55.8399, -7.2718) ccw
  line L266 (-56.547, -6.5647) -> (-54.6399, -4.6576)
  line L267 (-54.3399, -4.6576) -> (-54.6399, -4.6576)
  line L268 (-54.3399, -4.6576) -> (-54.0399, -4.6576)
  arc A107 (-51.8399, -7.2718) -> (-52.1328, -6.5647) centre (-52.8399, -7.2718) ccw
  line L269 (-52.1328, -6.5647) -> (-54.0399, -4.6576)
  arc A108 (-75.8328, -30.2647) -> (-75.1257, -30.5576) centre (-75.1257, -29.5576) ccw
  arc A109 (-75.1257, -25.5576) -> (-75.8328, -25.8505) centre (-75.1257, -26.5576) ccw
  line L270 (-75.8328, -30.2647) -> (-77.7399, -28.3576)
  line L271 (-75.8328, -25.8505) -> (-77.7399, -27.7576)
  line L272 (-77.7399, -28.0576) -> (-77.7399, -28.3576)
  line L273 (-77.7399, -28.0576) -> (-77.7399, -27.7576)
  line L274 (-75.1257, -25.5576) -> (-58.3541, -25.5576)
  line L275 (-58.3541, -30.5576) -> (-75.1257, -30.5576)
  arc A110 (-57.647, -25.8505) -> (-58.3541, -25.5576) centre (-58.3541, -26.5576) ccw
  line L276 (-57.647, -25.8505) -> (-55.7399, -27.7576)
  line L277 (-55.7399, -28.0576) -> (-55.7399, -27.7576)
  line L278 (-55.7399, -28.0576) -> (-55.7399, -28.3576)
  arc A111 (-58.3541, -30.5576) -> (-57.647, -30.2647) centre (-58.3541, -29.5576) ccw
  line L279 (-57.647, -30.2647) -> (-55.7399, -28.3576)
  arc A112 (-113.1328, 19.3353) -> (-112.4257, 19.0424) centre (-112.4257, 20.0424) ccw
  arc A113 (-112.4257, 24.0424) -> (-113.1328, 23.7495) centre (-112.4257, 23.0424) ccw
  line L280 (-113.1328, 19.3353) -> (-115.0399, 21.2424)
  line L281 (-113.1328, 23.7495) -> (-115.0399, 21.8424)
  line L282 (-115.0399, 21.5424) -> (-115.0399, 21.2424)
  line L283 (-115.0399, 21.5424) -> (-115.0399, 21.8424)
  line L284 (-112.4257, 24.0424) -> (-95.6541, 24.0424)
  line L285 (-95.6541, 19.0424) -> (-112.4257, 19.0424)
  arc A114 (-94.947, 23.7495) -> (-95.6541, 24.0424) centre (-95.6541, 23.0424) ccw
  line L286 (-94.947, 23.7495) -> (-93.0399, 21.8424)
  line L287 (-93.0399, 21.5424) -> (-93.0399, 21.8424)
  line L288 (-93.0399, 21.5424) -> (-93.0399, 21.2424)
  arc A115 (-95.6541, 19.0424) -> (-94.947, 19.3353) centre (-95.6541, 20.0424) ccw
  line L289 (-94.947, 19.3353) -> (-93.0399, 21.2424)
  arc A116 (-113.1328, -5.4647) -> (-112.4257, -5.7576) centre (-112.4257, -4.7576) ccw
  arc A117 (-112.4257, -0.7576) -> (-113.1328, -1.0505) centre (-112.4257, -1.7576) ccw
  line L290 (-113.1328, -5.4647) -> (-115.0399, -3.5576)
  line L291 (-113.1328, -1.0505) -> (-115.0399, -2.9576)
  line L292 (-115.0399, -3.2576) -> (-115.0399, -3.5576)
  line L293 (-115.0399, -3.2576) -> (-115.0399, -2.9576)
  line L294 (-112.4257, -0.7576) -> (-95.6541, -0.7576)
  line L295 (-95.6541, -5.7576) -> (-112.4257, -5.7576)
  arc A118 (-94.947, -1.0505) -> (-95.6541, -0.7576) centre (-95.6541, -1.7576) ccw
  line L296 (-94.947, -1.0505) -> (-93.0399, -2.9576)
  line L297 (-93.0399, -3.2576) -> (-93.0399, -2.9576)
  line L298 (-93.0399, -3.2576) -> (-93.0399, -3.5576)
  arc A119 (-95.6541, -5.7576) -> (-94.947, -5.4647) centre (-95.6541, -4.7576) ccw
  line L299 (-94.947, -5.4647) -> (-93.0399, -3.5576)
  arc A120 (-114.2328, 0.0495) -> (-113.9399, 0.7566) centre (-114.9399, 0.7566) ccw
  arc A121 (-118.9399, 0.7566) -> (-118.647, 0.0495) centre (-117.9399, 0.7566) ccw
  line L300 (-114.2328, 0.0495) -> (-116.1399, -1.8576)
  line L301 (-118.647, 0.0495) -> (-116.7399, -1.8576)
  line L302 (-116.4399, -1.8576) -> (-116.1399, -1.8576)
  line L303 (-116.4399, -1.8576) -> (-116.7399, -1.8576)
  line L304 (-118.9399, 0.7566) -> (-118.9399, 17.5282)
  line L305 (-113.9399, 17.5282) -> (-113.9399, 0.7566)
  arc A122 (-118.647, 18.2353) -> (-118.9399, 17.5282) centre (-117.9399, 17.5282) ccw
  line L306 (-118.647, 18.2353) -> (-116.7399, 20.1424)
  line L307 (-116.4399, 20.1424) -> (-116.7399, 20.1424)
  line L308 (-116.4399, 20.1424) -> (-116.1399, 20.1424)
  arc A123 (-113.9399, 17.5282) -> (-114.2328, 18.2353) centre (-114.9399, 17.5282) ccw
  line L309 (-114.2328, 18.2353) -> (-116.1399, 20.1424)
  arc A124 (-114.2328, -24.7505) -> (-113.9399, -24.0434) centre (-114.9399, -24.0434) ccw
  arc A125 (-118.9399, -24.0434) -> (-118.647, -24.7505) centre (-117.9399, -24.0434) ccw
  line L310 (-114.2328, -24.7505) -> (-116.1399, -26.6576)
  line L311 (-118.647, -24.7505) -> (-116.7399, -26.6576)
  line L312 (-116.4399, -26.6576) -> (-116.1399, -26.6576)
  line L313 (-116.4399, -26.6576) -> (-116.7399, -26.6576)
  line L314 (-118.9399, -24.0434) -> (-118.9399, -7.2718)
  line L315 (-113.9399, -7.2718) -> (-113.9399, -24.0434)
  arc A126 (-118.647, -6.5647) -> (-118.9399, -7.2718) centre (-117.9399, -7.2718) ccw
  line L316 (-118.647, -6.5647) -> (-116.7399, -4.6576)
  line L317 (-116.4399, -4.6576) -> (-116.7399, -4.6576)
  line L318 (-116.4399, -4.6576) -> (-116.1399, -4.6576)
  arc A127 (-113.9399, -7.2718) -> (-114.2328, -6.5647) centre (-114.9399, -7.2718) ccw
  line L319 (-114.2328, -6.5647) -> (-116.1399, -4.6576)
  arc A128 (-89.4328, 0.0495) -> (-89.1399, 0.7566) centre (-90.1399, 0.7566) ccw
  arc A129 (-94.1399, 0.7566) -> (-93.847, 0.0495) centre (-93.1399, 0.7566) ccw
  line L320 (-89.4328, 0.0495) -> (-91.3399, -1.8576)
  line L321 (-93.847, 0.0495) -> (-91.9399, -1.8576)
  line L322 (-91.6399, -1.8576) -> (-91.3399, -1.8576)
  line L323 (-91.6399, -1.8576) -> (-91.9399, -1.8576)
  line L324 (-94.1399, 0.7566) -> (-94.1399, 17.5282)
  line L325 (-89.1399, 17.5282) -> (-89.1399, 0.7566)
  arc A130 (-93.847, 18.2353) -> (-94.1399, 17.5282) centre (-93.1399, 17.5282) ccw
  line L326 (-93.847, 18.2353) -> (-91.9399, 20.1424)
  line L327 (-91.6399, 20.1424) -> (-91.9399, 20.1424)
  line L328 (-91.6399, 20.1424) -> (-91.3399, 20.1424)
  arc A131 (-89.1399, 17.5282) -> (-89.4328, 18.2353) centre (-90.1399, 17.5282) ccw
  line L329 (-89.4328, 18.2353) -> (-91.3399, 20.1424)
  arc A132 (-89.4328, -24.7505) -> (-89.1399, -24.0434) centre (-90.1399, -24.0434) ccw
  arc A133 (-94.1399, -24.0434) -> (-93.847, -24.7505) centre (-93.1399, -24.0434) ccw
  line L330 (-89.4328, -24.7505) -> (-91.3399, -26.6576)
  line L331 (-93.847, -24.7505) -> (-91.9399, -26.6576)
  line L332 (-91.6399, -26.6576) -> (-91.3399, -26.6576)
  line L333 (-91.6399, -26.6576) -> (-91.9399, -26.6576)
  line L334 (-94.1399, -24.0434) -> (-94.1399, -7.2718)
  line L335 (-89.1399, -7.2718) -> (-89.1399, -24.0434)
  arc A134 (-93.847, -6.5647) -> (-94.1399, -7.2718) centre (-93.1399, -7.2718) ccw
  line L336 (-93.847, -6.5647) -> (-91.9399, -4.6576)
  line L337 (-91.6399, -4.6576) -> (-91.9399, -4.6576)
  line L338 (-91.6399, -4.6576) -> (-91.3399, -4.6576)
  arc A135 (-89.1399, -7.2718) -> (-89.4328, -6.5647) centre (-90.1399, -7.2718) ccw
  line L339 (-89.4328, -6.5647) -> (-91.3399, -4.6576)
  arc A136 (-113.1328, -30.2647) -> (-112.4257, -30.5576) centre (-112.4257, -29.5576) ccw
  arc A137 (-112.4257, -25.5576) -> (-113.1328, -25.8505) centre (-112.4257, -26.5576) ccw
  line L340 (-113.1328, -30.2647) -> (-115.0399, -28.3576)
  line L341 (-113.1328, -25.8505) -> (-115.0399, -27.7576)
  line L342 (-115.0399, -28.0576) -> (-115.0399, -28.3576)
  line L343 (-115.0399, -28.0576) -> (-115.0399, -27.7576)
  line L344 (-112.4257, -25.5576) -> (-95.6541, -25.5576)
  line L345 (-95.6541, -30.5576) -> (-112.4257, -30.5576)
  arc A138 (-94.947, -25.8505) -> (-95.6541, -25.5576) centre (-95.6541, -26.5576) ccw
  line L346 (-94.947, -25.8505) -> (-93.0399, -27.7576)
  line L347 (-93.0399, -28.0576) -> (-93.0399, -27.7576)
  line L348 (-93.0399, -28.0576) -> (-93.0399, -28.3576)
  arc A139 (-95.6541, -30.5576) -> (-94.947, -30.2647) centre (-95.6541, -29.5576) ccw
  line L349 (-94.947, -30.2647) -> (-93.0399, -28.3576)
  arc A140 (92.3672, 19.3353) -> (93.0743, 19.0424) centre (93.0743, 20.0424) ccw
  arc A141 (93.0743, 24.0424) -> (92.3672, 23.7495) centre (93.0743, 23.0424) ccw
  line L350 (92.3672, 19.3353) -> (90.4601, 21.2424)
  line L351 (92.3672, 23.7495) -> (90.4601, 21.8424)
  line L352 (90.4601, 21.5424) -> (90.4601, 21.2424)
  line L353 (90.4601, 21.5424) -> (90.4601, 21.8424)
  line L354 (93.0743, 24.0424) -> (109.8459, 24.0424)
  line L355 (109.8459, 19.0424) -> (93.0743, 19.0424)
  arc A142 (110.553, 23.7495) -> (109.8459, 24.0424) centre (109.8459, 23.0424) ccw
  line L356 (110.553, 23.7495) -> (112.4601, 21.8424)
  line L357 (112.4601, 21.5424) -> (112.4601, 21.8424)
  line L358 (112.4601, 21.5424) -> (112.4601, 21.2424)
  arc A143 (109.8459, 19.0424) -> (110.553, 19.3353) centre (109.8459, 20.0424) ccw
  line L359 (110.553, 19.3353) -> (112.4601, 21.2424)
  arc A144 (92.3672, -5.4647) -> (93.0743, -5.7576) centre (93.0743, -4.7576) ccw
  arc A145 (93.0743, -0.7576) -> (92.3672, -1.0505) centre (93.0743, -1.7576) ccw
  line L360 (92.3672, -5.4647) -> (90.4601, -3.5576)
  line L361 (92.3672, -1.0505) -> (90.4601, -2.9576)
  line L362 (90.4601, -3.2576) -> (90.4601, -3.5576)
  line L363 (90.4601, -3.2576) -> (90.4601, -2.9576)
  line L364 (93.0743, -0.7576) -> (109.8459, -0.7576)
  line L365 (109.8459, -5.7576) -> (93.0743, -5.7576)
  arc A146 (110.553, -1.0505) -> (109.8459, -0.7576) centre (109.8459, -1.7576) ccw
  line L366 (110.553, -1.0505) -> (112.4601, -2.9576)
  line L367 (112.4601, -3.2576) -> (112.4601, -2.9576)
  line L368 (112.4601, -3.2576) -> (112.4601, -3.5576)
  arc A147 (109.8459, -5.7576) -> (110.553, -5.4647) centre (109.8459, -4.7576) ccw
  line L369 (110.553, -5.4647) -> (112.4601, -3.5576)
  arc A148 (91.2672, 0.0495) -> (91.5601, 0.7566) centre (90.5601, 0.7566) ccw
  arc A149 (86.5601, 0.7566) -> (86.853, 0.0495) centre (87.5601, 0.7566) ccw
  line L370 (91.2672, 0.0495) -> (89.3601, -1.8576)
  line L371 (86.853, 0.0495) -> (88.7601, -1.8576)
  line L372 (89.0601, -1.8576) -> (89.3601, -1.8576)
  line L373 (89.0601, -1.8576) -> (88.7601, -1.8576)
  line L374 (86.5601, 0.7566) -> (86.5601, 17.5282)
  line L375 (91.5601, 17.5282) -> (91.5601, 0.7566)
  arc A150 (86.853, 18.2353) -> (86.5601, 17.5282) centre (87.5601, 17.5282) ccw
  line L376 (86.853, 18.2353) -> (88.7601, 20.1424)
  line L377 (89.0601, 20.1424) -> (88.7601, 20.1424)
  line L378 (89.0601, 20.1424) -> (89.3601, 20.1424)
  arc A151 (91.5601, 17.5282) -> (91.2672, 18.2353) centre (90.5601, 17.5282) ccw
  line L379 (91.2672, 18.2353) -> (89.3601, 20.1424)
  arc A152 (91.2672, -24.7505) -> (91.5601, -24.0434) centre (90.5601, -24.0434) ccw
  arc A153 (86.5601, -24.0434) -> (86.853, -24.7505) centre (87.5601, -24.0434) ccw
  line L380 (91.2672, -24.7505) -> (89.3601, -26.6576)
  line L381 (86.853, -24.7505) -> (88.7601, -26.6576)
  line L382 (89.0601, -26.6576) -> (89.3601, -26.6576)
  line L383 (89.0601, -26.6576) -> (88.7601, -26.6576)